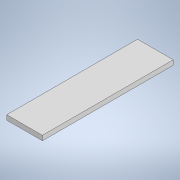
# Autodesk Inventor part: FP Spoilers (2)
Saved by Autodesk Inventor 2020 (Build 240168000, 168)
## iProperties
Created: 2021-04-23
Part Number: FP Spoilers (2)
Material: Generic
Document SubType Name: Modeling
Designer: austi
Density: 1 g/cm^3
Appearance: Default
Author: austi
Autodesk Inventor part; units mm, degrees
ref_plane "YZ Plane" through (0, 0, 0) normal (1, 0, 0) x (0, 1, 0)
ref_plane "XZ Plane" through (0, 0, 0) normal (0, 1, 0) x (-1, 0, 0)
ref_plane "XY Plane" through (0, 0, 0) normal (0, 0, 1) x (1, 0, 0)
sketch "Sketch1" plane through (0, 0, 0) normal (0, 1, 0) x (-1, 0, 0)
  line L0 (7.5, 27.5) -> (-7.5, 27.5)
  line L1 (-7.5, 27.5) -> (-7.5, -27.5)
  line L2 (-7.5, -27.5) -> (7.5, -27.5)
  line L3 (7.5, -27.5) -> (7.5, 27.5)
  point P0 (0, 0)
  point P1 (0, 27.5)
  point P2 (7.5, 0)
  dimension "d0" = 15
  dimension "d1" = 55
  constraints: 8 end point, 2 midpoint, 2 parallel, 1 horizontal, 1 horizontal alignment, 1 perpendicular, 1 vertical alignment
  measures "d0" distance of L2.end L1.end
  measures "d1" distance of L1.end L0.end
extrude "Extrusion1" add sketch "Sketch1" along normal blind 2
body "Solid1"
